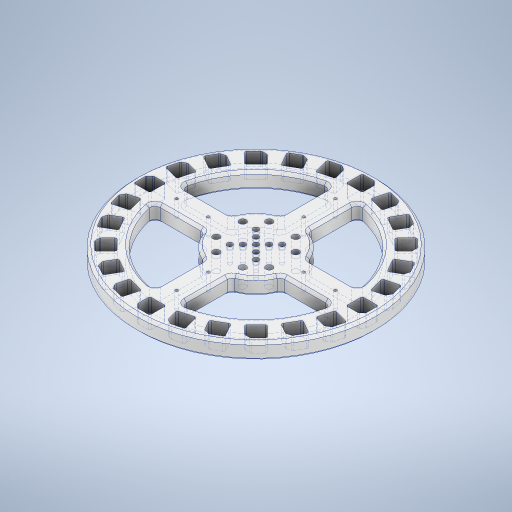
# Autodesk Inventor part: Sample Tray Mass Delete
Saved by Autodesk Inventor 2024 (Build 280153000, 153)
## iProperties
Created: 2023-10-26
Part Number: Sample Tray Mass Delete
Material: Aluminum 6061
Document SubType Name: Modeling
Designer: Besher
Density: 2.7 g/cm^3
Appearance: Aluminum - Flat
Mass: 7795.53 g
Surface Area: 4067 cm^2
Volume: 2887.23 cm^3
Author: Besher
Autodesk Inventor part; units mm, degrees
sketch "Sketch1" plane through (0, 0, 0) normal (0, 1, 0) x (-1, 0, 0)
  circle A0 centre (0, 0) radius 228.6
  dimension "d0" = 457.2
  constraints: 1 centre point
  measures "d0" diameter of A0
extrude "Extrusion1" add sketch "Sketch1" along normal blind 38.1
sketch "Sketch3" plane through (0, 38.1, 0) normal (0, 1, 0) x (1, 0, 0)
  circle A0 centre (0, 0) radius 228.6 projected
  line L0 (0, 228.6) -> (0, 203.2)
  line L1 (-15.367, 218.567) -> (15.367, 218.567)
  line L2 (15.367, 218.567) -> (15.367, 187.833)
  line L3 (15.367, 187.833) -> (-15.367, 187.833)
  line L4 (-15.367, 187.833) -> (-15.367, 218.567)
  line L5 (-15.367, 218.567) -> (15.367, 187.833) construction
  line L6 (15.367, 218.567) -> (-15.367, 187.833) construction
  dimension "d14" = 25.4
  dimension "d15" = 30.734
  dimension "d16" = 30.734
  constraints: 14 end point, 2 midpoint, 2 parallel, 1 horizontal, 1 perpendicular, 1 vertical, 1 vertical alignment, 1 other
  measures "d14" distance of L0.start L0.end
  measures "d15" distance of L2.end L3.end
  measures "d16" distance of L1.end L2.end
extrude "Extrusion2" cut sketch "Sketch3" against normal blind 25.4 contours L1 L2 L3 L4
sketch "Sketch4" plane through (0, 12.7, 0) normal (0, 1, 0) x (1, 0, 0)
  line L0 (15.367, 218.567) -> (15.367, 187.833) projected
  line L1 (15.367, 218.567) -> (7.747, 218.567)
  line L2 (-15.367, 218.567) -> (15.367, 218.567) projected
  line L3 (15.367, 218.567) -> (15.367, 210.947)
  line L4 (15.367, 210.947) -> (7.747, 218.567)
  point P0 (0, 0)
  dimension "d19" = 7.62
  dimension "d20" = 7.62
  constraints: 6 end point, 2 point on line
  measures "d19" distance of L0.start L1.end
  measures "d20" distance of L0.start L3.end
extrude "Extrusion3" add sketch "Sketch4" along normal up to surface (25.4 mm away)
pattern_circular "Circular Pattern1" count 24 over 360 about axis through (0, 0, 0) along (0, 1, 0) of "Extrusion2", "Extrusion3"
sketch "Sketch7" plane through (0, 0, 0) normal (0, 0, 1) x (1, 0, 0)
  line L0 (228.6, 0) -> (-228.6, 0) projected
  line L1 (-228.6, 0) -> (-228.6, 38.1) projected
  line L2 (228.6, 0) -> (-228.6, 0)
  line L3 (-228.6, 0) -> (-228.6, 6.35)
  line L4 (-228.6, 6.35) -> (228.6, 6.35)
  line L5 (228.6, 6.35) -> (228.6, 0)
  point P0 (0, 0)
  dimension "d49" = 6.35
  constraints: 8 end point, 2 parallel, 1 horizontal, 1 perpendicular, 1 point on line
  measures "d49" distance between parallel lines of L0 L4
extrude "Extrusion5" cut sketch "Sketch7" along normal through all both and the other way through all
ref_plane "Work Plane2" through (0, 38.1, -187.833) normal (-1, 0, 0) x (0, -1, 0)
sketch "Sketch29" plane through (0, 38.1, 0) normal (0, 1, 0) x (1, 0, 0)
  circle A0 centre (-12.5, 12.5) radius 2.5
  circle A1 centre (-12.5, 12.5) radius 3.5052
  circle A2 centre (-25, 25) radius 3.5052
  circle A3 centre (-25, 25) radius 2.5
  circle A4 centre (-12.5, -12.5) radius 3.5052
  circle A5 centre (-12.5, -12.5) radius 2.5
  circle A6 centre (-25, -25) radius 3.5052
  circle A7 centre (-25, -25) radius 2.5
  circle A8 centre (25, -25) radius 3.5052
  circle A9 centre (25, -25) radius 2.5
  circle A10 centre (12.5, -12.5) radius 2.5
  circle A11 centre (12.5, -12.5) radius 3.5052
  circle A12 centre (12.5, 12.5) radius 3.5052
  circle A13 centre (12.5, 12.5) radius 2.5
  circle A14 centre (25, 25) radius 3.5052
  circle A15 centre (25, 25) radius 2.5
  circle A16 centre (0, 0) radius 3.5052
  point P0 (-3.3774, 2.1461)
  dimension "d102" = 17.6777
  dimension "d103" = 17.6777
  dimension "d104" = 17.6777
  dimension "d105" = 17.6777
  dimension "d106" = 17.6777
  dimension "d107" = 17.6777
  dimension "d108" = 17.6777
  dimension "d109" = 17.6777
  dimension "d111" = 7.0104
  dimension "d112" = 7.0104
  dimension "d190" = 7.0104
  constraints: 17 centre point, 9 coincident, 7 equal radius
  measures "d102" distance of A1.centre A2.centre
  measures "d103" distance of A16.centre A1.centre
  measures "d104" distance of A13.centre A16.centre
  measures "d105" distance of A14.centre A13.centre
  measures "d106" distance of A11.centre A16.centre
  measures "d107" distance of A8.centre A11.centre
  measures "d108" distance of A16.centre A5.centre
  measures "d109" distance of A5.centre A7.centre
  measures "d111" diameter of A16
  measures "d112" diameter of A2
  measures "d190" diameter of A1
extrude "Extrusion9" cut sketch "Sketch29" against normal up to surface (31.75 mm away) contours A0 | A1 | A2 | A3 | A4 | A5 | A6 | A7 | A8 | A9 | A10 | A11 | A12 | A13 | A14 | A15 | A16
sketch "Sketch33" plane through (0, 38.1, 0) normal (0, 1, 0) x (1, 0, 0)
  circle A0 centre (50.6, -25.3) radius 6.35
  circle A1 centre (50.6, 25.3) radius 6.35
  circle A2 centre (-50.6, -25.3) radius 6.35
  circle A3 centre (-50.6, 25.3) radius 6.35
  line L0 (50.6, 25.3) -> (-50.6, -25.3)
  line L1 (-50.6, 25.3) -> (50.6, -25.3)
  circle A4 centre (0, 0) radius 3.5052 projected
  line L2 (0, 0) -> (-50.6, 0)
  circle A5 centre (-25.3, 50.5968) radius 6.35
  circle A6 centre (25.2984, 50.5968) radius 6.35
  circle A7 centre (25.2984, -50.5968) radius 6.35
  line L3 (0, 0) -> (-25.3, 0)
  circle A8 centre (-25.3, -50.5968) radius 6.35
  point P0 (138.0178, 18.4089)
  point P1 (50.6, 25.3)
  dimension "d133" = 12.7
  dimension "d134" = 53.13
  dimension "d135" = 0
  dimension "d136" = 45.258
  dimension "d137" = 45.258
  dimension "d138" = 45.258
  dimension "d139" = 45.258
  dimension "d140" = 0
  dimension "d141" = 45.258
  dimension "d147" = 25.3
  dimension "d148" = 12.7
  dimension "d151" = 12.7
  dimension "d153" = 12.7
  dimension "d154" = 12.7
  constraints: 8 centre point, 8 end point, 3 equal radius, 2 horizontal, 1 coincident, 1 midpoint
  measures "d133" diameter of A1
  measures "d134" angle of L0 L1
  measures "d135" distance from line of point (50.6, 25.3) L0
  measures "d136" distance from line of point (50.6, 25.3) L1
  measures "d137" distance from line of point (138.018, 18.409) L0
  measures "d138" distance from line of L0.start L1
  measures "d139" distance from line of L1.end L0
  measures "d140" distance from line of point (0, 0) L0
  measures "d141" distance from line of L0.end L1
  measures "d147" distance of L2.end L1.start
  measures "d148" diameter of A5
  measures "d151" diameter of A6
  measures "d153" diameter of A7
  measures "d154" diameter of A8
extrude "Extrusion11" cut sketch "Sketch33" against normal through all contours A0 | A2 | A3 | A1
ref_plane "Work Plane3" through (0, 38.1, 0) normal (0, 1, 0) x (1, 0, 0)
sketch "Sketch36" plane through (0, 38.1, 0) normal (0, 1, 0) x (1, 0, 0)
  circle A0 centre (-25.2992, 50.5968) radius 6.35
  circle A1 centre (25.2992, 50.5968) radius 6.35
  circle A2 centre (25.2992, -50.5968) radius 6.35
  circle A3 centre (-25.2992, -50.5968) radius 6.35
  line L0 (-25.2992, -50.5968) -> (25.2992, 50.5968) construction
  line L1 (-25.2992, 50.5968) -> (25.2992, -50.5968) construction
  point P0 (0, 0)
  point P1 (0, 0)
  dimension "d161" = 12.7
  dimension "d162" = 12.7
  dimension "d163" = 12.7
  dimension "d164" = 12.7
  dimension "d165" = 126.868
  dimension "d168" = 45.2563
  dimension "d169" = 45.2563
  dimension "d170" = 0
  dimension "d171" = 45.2563
  constraints: 4 centre point, 4 end point, 1 coincident, 1 midpoint
  measures "d161" diameter of A0
  measures "d162" diameter of A1
  measures "d163" diameter of A2
  measures "d164" diameter of A3
  measures "d165" angle of L0 L1
  measures "d168" distance from line of L0.end L1
  measures "d169" distance from line of L1.end L0
  measures "d170" distance from line of point (0, 0) L0
  measures "d171" distance from line of L0.start L1
extrude "Extrusion12" cut sketch "Sketch36" against normal through all
fillet "Fillet3" radius 3.175 35 edges at (-115.9926, 25.4, 185.4111) (-118.7817, 25.4, 175.002) (-95.9753, 25.4, 196.9681) (-80.6083, 25.4, 170.3516) (-107.2247, 25.4, 154.9846) (-143.6841, 25.4, 121.9519) (-121.9519, 25.4, 143.6841) (-143.6841, 25.4, 165.4163) (-160.0282, 25.4, 149.0723) (-160.0282, 25.4, 138.2959) (-181.6011, 25.4, 122.5917) (-193.1581, 25.4, 102.5744) (-190.369, 25.4, 92.1653) (-154.9846, 25.4, 107.2247) (-170.3516, 25.4, 80.6083) (-207.1422, 25.4, 71.4127) (-213.1246, 25.4, 49.0863) (-207.7364, 25.4, 39.7537) (-177.4555, 25.4, 63.4581) (-185.41, 25.4, 33.7714) (-218.567, 25.4, 15.367) (-187.833, 25.4, 15.367) (-187.833, 25.4, -15.367) (-210.947, 25.4, -15.367) (-218.567, 25.4, -7.747) (-209.1144, 25.4, -64.0523) (-199.7819, 25.4, -69.4405) (-177.4555, 25.4, -63.4581) (-185.41, 25.4, -33.7714) (-215.0968, 25.4, -41.7259) (-196.9681, 25.4, -95.9753) (-170.3516, 25.4, -80.6083) (-175.002, 25.4, -118.7817) (-185.4111, 25.4, -115.9926) (-154.9846, 25.4, -107.2247)
fillet "Fillet4" radius 3.175 52 edges at (-149.0723, 25.4, -160.0282) (-138.2959, 25.4, -160.0282) (-165.4163, 25.4, -143.6841) (-143.6841, 25.4, -121.9519) (-121.9519, 25.4, -143.6841) (-80.6083, 25.4, -170.3516) (-107.2247, 25.4, -154.9846) (-122.5917, 25.4, -181.6011) (-102.5744, 25.4, -193.1581) (-92.1653, 25.4, -190.369) (-71.4127, 25.4, -207.1422) (-63.4581, 25.4, -177.4555) (-49.0863, 25.4, -213.1246) (-39.7537, 25.4, -207.7364) (-33.7714, 25.4, -185.41) (-15.367, 25.4, -187.833) (-15.367, 25.4, -218.567) (7.747, 25.4, -218.567) (15.367, 25.4, -210.947) (15.367, 25.4, -187.833) (41.7259, 25.4, -215.0968) (33.7714, 25.4, -185.41) (63.4581, 25.4, -177.4555) (69.4405, 25.4, -199.7819) (64.0523, 25.4, -209.1144) (107.2247, 25.4, -154.9846) (80.6083, 25.4, -170.3516) (95.9753, 25.4, -196.9681) (115.9926, 25.4, -185.4111) (118.7817, 25.4, -175.002) (121.9519, 25.4, -143.6841) (143.6841, 25.4, -165.4163) (160.0282, 25.4, -149.0723) (160.0282, 25.4, -138.2959) (143.6841, 25.4, -121.9519) (181.6011, 25.4, -122.5917) (154.9846, 25.4, -107.2247) (170.3516, 25.4, -80.6083) (193.1581, 25.4, -102.5744) (190.369, 25.4, -92.1653) (177.4555, 25.4, -63.4581) (185.41, 25.4, -33.7714) (213.1246, 25.4, -49.0863) (207.7364, 25.4, -39.7537) (207.1422, 25.4, -71.4127) (187.833, 25.4, 15.367) (187.833, 25.4, -15.367) (210.947, 25.4, 15.367) (218.567, 25.4, 7.747) (218.567, 25.4, -15.367) (177.4555, 25.4, 63.4581) (185.41, 25.4, 33.7714)
fillet "Fillet5" radius 3.175 33 edges at (199.7819, 25.4, 69.4405) (209.1144, 25.4, 64.0523) (215.0968, 25.4, 41.7259) (154.9846, 25.4, 107.2247) (175.002, 25.4, 118.7817) (185.4111, 25.4, 115.9926) (170.3516, 25.4, 80.6083) (196.9681, 25.4, 95.9753) (138.2959, 25.4, 160.0282) (121.9519, 25.4, 143.6841) (149.0723, 25.4, 160.0282) (165.4163, 25.4, 143.6841) (143.6841, 25.4, 121.9519) (80.6083, 25.4, 170.3516) (92.1653, 25.4, 190.369) (107.2247, 25.4, 154.9846) (122.5917, 25.4, 181.6011) (102.5744, 25.4, 193.1581) (33.7714, 25.4, 185.41) (63.4581, 25.4, 177.4555) (39.7537, 25.4, 207.7364) (49.0863, 25.4, 213.1246) (71.4127, 25.4, 207.1422) (-15.367, 25.4, 187.833) (-15.367, 25.4, 210.947) (15.367, 25.4, 187.833) (15.367, 25.4, 218.567) (-7.747, 25.4, 218.567) (-63.4581, 25.4, 177.4555) (-33.7714, 25.4, 185.41) (-69.4405, 25.4, 199.7819) (-64.0523, 25.4, 209.1144) (-41.7259, 25.4, 215.0968)
ref_plane "Work Plane9" through (0, 38.1, 0) normal (0, 1, 0) x (1, 0, 0)
sketch "Sketch39" plane through (0, 38.1, 0) normal (0, 1, 0) x (1, 0, 0)
  circle A0 centre (0, 0) radius 5.207
  circle A1 centre (-25, -25) radius 3.5052 projected
  circle A2 centre (-12.5, -12.5) radius 3.5052 projected
  circle A3 centre (-12.5, 12.5) radius 3.5052 projected
  circle A4 centre (-25, 25) radius 3.5052 projected
  circle A5 centre (12.5, 12.5) radius 3.5052 projected
  circle A6 centre (25, 25) radius 3.5052 projected
  circle A7 centre (12.5, -12.5) radius 3.5052 projected
  circle A8 centre (25, -25) radius 3.5052 projected
  circle A9 centre (12.5, -12.5) radius 5.207
  circle A10 centre (25, -25) radius 5.207
  circle A11 centre (12.5, 12.5) radius 5.207
  circle A12 centre (25, 25) radius 5.207
  circle A13 centre (-12.5, 12.5) radius 5.207
  circle A14 centre (-25, 25) radius 5.207
  circle A15 centre (-12.5, -12.5) radius 5.207
  circle A16 centre (-25, -25) radius 5.207
  dimension "d177" = 10.414
  dimension "d178" = 10.414
  dimension "d179" = 10.414
  dimension "d180" = 10.414
  dimension "d181" = 10.414
  dimension "d184" = 10.414
  dimension "d185" = 10.414
  dimension "d186" = 10.414
  dimension "d187" = 10.414
  constraints: 9 centre point, 9 coincident
  measures "d177" diameter of A0
  measures "d178" diameter of A9
  measures "d179" diameter of A10
  measures "d180" diameter of A13
  measures "d181" diameter of A14
  measures "d184" diameter of A11
  measures "d185" diameter of A12
  measures "d186" diameter of A16
  measures "d187" diameter of A15
extrude "Extrusion13" cut sketch "Sketch39" against normal blind 6.604 contours A0 | A1 | A2 | A3 | A4 | A5 | A6 | A7 | A8 | A9 | A10 | A11 | A12 | A13 | A14 | A15 | A16
ref_plane "Work Plane5" through (0, 38.1, 0) normal (0, 1, 0) x (1, 0, 0)
sketch "Sketch42" plane through (0, 38.1, 0) normal (0, 1, 0) x (1, 0, 0)
  circle A0 centre (0, 0) radius 3.5052 projected
  circle A1 centre (0, 0) radius 77.7875
  circle A2 centre (0, 0) radius 171.45
  line L0 (-73.5237, 25.4) -> (-169.5581, 25.4)
  line L1 (-169.5581, -25.4) -> (-73.5237, -25.4)
  line L2 (0, 0) -> (-217.4875, 0) construction
  line L3 (25.4, 73.5237) -> (25.4, 169.5581)
  line L4 (-25.4, 169.5581) -> (-25.4, 73.5237)
  line L5 (-25.4, -73.5237) -> (-25.4, -169.5581)
  line L6 (25.4, -169.5581) -> (25.4, -73.5237)
  line L7 (73.5237, -25.4) -> (169.5581, -25.4)
  line L8 (169.5581, 25.4) -> (73.5237, 25.4)
  point P0 (-25.4, 73.5237)
  dimension "d191" = 25.4
  dimension "d192" = 25.4
  constraints: 18 end point, 4 parallel, 2 coincident, 2 horizontal, 6 other
  measures "d191" distance between parallel lines of L2 L0
  measures "d192" distance between parallel lines of L2 L1
extrude "Extrusion14" cut sketch "Sketch42" against normal through all contours A1 L3 A2 L8 | L7 A2 L6 A1 | A1 L0 A2 L4 | L5 A2 L1 A1
ref_plane "Work Plane8" through (0, 38.1, 0) normal (0, 1, 0) x (1, 0, 0)
sketch "Sketch43" plane through (0, 38.1, 0) normal (0, 1, 0) x (1, 0, 0)
  circle A0 centre (0, 0) radius 3.5052 construction
  line L0 (0, 0) -> (-236.5375, 0) construction
  line L1 (0, 0) -> (0, 254) construction
  circle A1 centre (-151.7781, 0) radius 2.54
  circle A2 centre (-91.3037, 0) radius 2.54
  line L2 (-73.5237, 25.4) -> (-73.5237, -25.4) construction
  arc A3 (-169.5581, -25.4) -> (-25.4, -169.5581) centre (0, 0) ccw construction
  line L3 (-169.5581, -25.4) -> (-169.5581, 25.4) construction
  circle A4 centre (0, 151.7781) radius 2.54
  circle A5 centre (0, 91.3037) radius 2.54
  circle A6 centre (151.7781, 0) radius 2.54
  circle A7 centre (91.3037, 0) radius 2.54
  circle A8 centre (0, -91.3037) radius 2.54
  circle A9 centre (0, -151.7781) radius 2.54
  dimension "d195" = 5.08
  dimension "d196" = 5.08
  dimension "d197" = 17.78
  dimension "d198" = 17.78
  dimension "d199" = 5.08
  dimension "d200" = 5.08
  dimension "d201" = 5.08
  dimension "d202" = 5.08
  dimension "d203" = 5.08
  dimension "d204" = 5.08
  constraints: 8 centre point, 8 end point, 3 vertical, 2 point on line, 1 horizontal
  measures "d195" diameter of A1
  measures "d196" diameter of A2
  measures "d197" distance from line of L3 A1.centre
  measures "d198" distance from line of L2 A2.centre
  measures "d199" diameter of A4
  measures "d200" diameter of A5
  measures "d201" diameter of A6
  measures "d202" diameter of A7
  measures "d203" diameter of A9
  measures "d204" diameter of A8
extrude "Extrusion15" cut sketch "Sketch43" against normal up to surface (31.75 mm away)
thread "Thread1" size "1/4-20 UNC" class "2B" standard "ANSI Unified Screw Threads" full length
fillet "Fillet6" radius 9.525 8 edges at (25.4, 22.225, 73.5237) (73.5237, 22.225, 25.4) (73.5237, 22.225, -25.4) (25.4, 22.225, -73.5237) (-25.4, 22.225, -73.5237) (-73.5237, 22.225, -25.4) (-25.4, 22.225, 73.5237) (-73.5237, 22.225, 25.4)
fillet "Fillet7" radius 9.525 8 edges at (25.4, 22.225, 169.5581) (169.5581, 22.225, 25.4) (169.5581, 22.225, -25.4) (25.4, 22.225, -169.5581) (-25.4, 22.225, -169.5581) (-169.5581, 22.225, -25.4) (-169.5581, 22.225, 25.4) (-25.4, 22.225, 169.5581)
chamfer "Chamfer2" distance 5.08 angle 45 66 edges at (228.6, 38.1, 0) (-121.2335, 38.1, 121.2335) (-165.5398, 38.1, 28.9602) (-119.0685, 38.1, 25.4) (-74.8062, 38.1, 26.9558) (-55.0041, 38.1, 55.0041) (-26.9558, 38.1, 74.8062) (-25.4, 38.1, 119.0685) (-28.9602, 38.1, 165.5398) (-119.0685, 38.1, -25.4) (-165.5398, 38.1, -28.9602) (-121.2335, 38.1, -121.2335) (-28.9602, 38.1, -165.5398) (-25.4, 38.1, -119.0685) (-26.9558, 38.1, -74.8062) (-55.0041, 38.1, -55.0041) (-74.8062, 38.1, -26.9558) (25.4, 38.1, 119.0685) (26.9558, 38.1, 74.8062) (55.0041, 38.1, 55.0041) (74.8062, 38.1, 26.9558) (119.0685, 38.1, 25.4) (165.5398, 38.1, 28.9602) (121.2335, 38.1, 121.2335) (28.9602, 38.1, 165.5398) (55.0041, 38.1, -55.0041) (26.9558, 38.1, -74.8062) (25.4, 38.1, -119.0685) (28.9602, 38.1, -165.5398) (121.2335, 38.1, -121.2335) (165.5398, 38.1, -28.9602) (119.0685, 38.1, -25.4) (74.8062, 38.1, -26.9558) (228.6, 6.35, 0) (119.0685, 6.35, 25.4) (74.8062, 6.35, 26.9558) (55.0041, 6.35, 55.0041) (26.9558, 6.35, 74.8062) (25.4, 6.35, 119.0685) (28.9602, 6.35, 165.5398) (121.2335, 6.35, 121.2335) (165.5398, 6.35, 28.9602) (119.0685, 6.35, -25.4) (165.5398, 6.35, -28.9602) (121.2335, 6.35, -121.2335) (28.9602, 6.35, -165.5398) (25.4, 6.35, -119.0685) (26.9558, 6.35, -74.8062) (55.0041, 6.35, -55.0041) (74.8062, 6.35, -26.9558) (-55.0041, 6.35, -55.0041) (-26.9558, 6.35, -74.8062) (-25.4, 6.35, -119.0685) (-28.9602, 6.35, -165.5398) (-121.2335, 6.35, -121.2335) (-165.5398, 6.35, -28.9602) (-119.0685, 6.35, -25.4) (-74.8062, 6.35, -26.9558) (-55.0041, 6.35, 55.0041) (-74.8062, 6.35, 26.9558) (-119.0685, 6.35, 25.4) (-165.5398, 6.35, 28.9602) (-121.2335, 6.35, 121.2335) (-28.9602, 6.35, 165.5398) (-25.4, 6.35, 119.0685) (-26.9558, 6.35, 74.8062)
sketch "Sketch44" plane through (0, 0, 0) normal (0, 0, 1) x (1, 0, 0)
  point P0 (0, 0)
body "Solid1"
